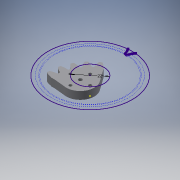
# Autodesk Inventor part: ENGE
Saved by Autodesk Inventor 2017 (Build 210142000, 142)
## iProperties
Created: 2018-01-13
Part Number: ENGE
Material: Generic
Document SubType Name: Modeling
Designer: Thomas
Density: 1 g/cm^3
Appearance: Default
Author: Thomas
Autodesk Inventor part; units mm, degrees
ref_plane "YZ Plane" through (0, 0, 0) normal (1, 0, 0) x (0, 1, 0)
ref_plane "XZ Plane" through (0, 0, 0) normal (0, 1, 0) x (-1, 0, 0)
ref_plane "XY Plane" through (0, 0, 0) normal (0, 0, 1) x (1, 0, 0)
sketch "Sketch1" plane through (0, 0, 0) normal (0, 0, 1) x (1, 0, 0)
  spline S0 degree 3 poles (-3.069, 32.857) (-2.9961, 32.7532) (-2.8503, 32.5455) (-2.641, 32.2277) (-2.4393, 31.9049) (-2.2462, 31.577) (-2.0623, 31.2438) (-1.8883, 30.9052) (-1.7251, 30.5614) (-1.5739, 30.2121) (-1.4358, 29.8574) (-1.3139, 29.4969) (-1.2064, 29.1316) (-1.1476, 28.8193) (-1.0633, 28.5794) (-0.9771, 28.4092) (-0.8642, 28.2551) (-0.725, 28.1239) (-0.5884, 28.0413) (-0.471, 27.9927) (-0.379, 27.968) (-0.2855, 27.9491) (-0.1585, 27.9444) (0, 27.9474) (0.1585, 27.9444) (0.2855, 27.9491) (0.379, 27.968) (0.471, 27.9927) (0.5884, 28.0413) (0.725, 28.1239) (0.8642, 28.2551) (0.9771, 28.4092) (1.0633, 28.5794) (1.1476, 28.8193) (1.2064, 29.1316) (1.3139, 29.4969) (1.4358, 29.8574) (1.5739, 30.2121) (1.7251, 30.5614) (1.8883, 30.9052) (2.0623, 31.2438) (2.2462, 31.577) (2.4393, 31.9049) (2.641, 32.2277) (2.8503, 32.5455) (2.9961, 32.7532) (3.069, 32.857) knots 0 0 0 0 0.038054 0.076108 0.114163 0.152217 0.190271 0.228324 0.266378 0.304431 0.342484 0.380536 0.418586 0.456634 0.47565 0.49466 0.513668 0.532673 0.551678 0.561193 0.570705 0.580215 0.589727 0.608754 0.627782 0.637294 0.646804 0.656316 0.66583 0.684836 0.703841 0.722849 0.741859 0.760875 0.798923 0.836973 0.875025 0.913077 0.95113 0.989184 1.027238 1.065292 1.103346 1.1414 1.179454 1.217508 1.217508 1.217508 1.217508
  circle A0 centre (0, 0) radius 27.9462 construction
  circle A1 centre (0, 0) radius 28.5432 construction
  circle A2 centre (0, 0) radius 30.375 construction
  circle A3 centre (0, 0) radius 33
  circle A4 centre (0, 0) radius 11
  point P0 (-2.8519, 32.5444)
  point P1 (-2.6423, 32.2269)
  point P2 (-2.4407, 31.9041)
  point P3 (-2.2477, 31.5761)
  point P4 (-2.0639, 31.2429)
  point P5 (-1.8901, 30.9044)
  point P6 (-1.7271, 30.5605)
  point P7 (-1.5761, 30.2112)
  point P8 (-1.4385, 29.8564)
  point P9 (-1.3163, 29.4961)
  point P10 (-1.2126, 29.13)
  point P11 (-1.1234, 28.7601)
  point P12 (-1.0595, 28.581)
  point P13 (-0.9726, 28.4119)
  point P14 (-0.8598, 28.2589)
  point P15 (-0.7209, 28.1293)
  point P16 (-0.5584, 28.0306)
  point P17 (-0.4703, 27.9947)
  point P18 (-0.3787, 27.969)
  point P19 (-0.2852, 27.9516)
  point P20 (-0.1903, 27.9462)
  point P21 (0, 27.9462)
  point P22 (0.1903, 27.9462)
  point P23 (0.2852, 27.9516)
  point P24 (0.3787, 27.969)
  point P25 (0.4703, 27.9947)
  point P26 (0.5584, 28.0306)
  point P27 (0.7209, 28.1293)
  point P28 (0.8598, 28.2589)
  point P29 (0.9726, 28.4119)
  point P30 (1.0595, 28.581)
  point P31 (1.1234, 28.7601)
  point P32 (1.2126, 29.13)
  point P33 (1.3163, 29.4961)
  point P34 (1.4385, 29.8564)
  point P35 (1.5761, 30.2112)
  point P36 (1.7271, 30.5605)
  point P37 (1.8901, 30.9044)
  point P38 (2.0639, 31.2429)
  point P39 (2.2477, 31.5761)
  point P40 (2.4407, 31.9041)
  point P41 (2.6423, 32.2269)
  point P42 (2.8519, 32.5444)
  dimension "d23" = 22
  constraints: 5 centre point, 2 point on circle, 1 coincident, 95 other
  measures "d23" diameter of A4
extrude "Extrusion1" add sketch "Sketch1" against normal blind 20 contours A3 S0 | S0 A3 | A4
extrude "Extrusion2" cut sketch "Sketch1" against normal blind 26.5 contours A3 S0 picked at (-0.225, 31.2542)
pattern_circular "Réseau circulaire1" count 26 over 360 about axis through (0, 0, -10) along (0, 0, 1) of "Extrusion2"
sketch "Esquisse2" plane through (0, 0, 0) normal (0, 0, 1) x (1, 0, 0)
  spline S0 degree 3 poles (28.7842, 16.1392) (28.6573, 16.1402) (28.4036, 16.1422) (28.0231, 16.1339) (27.6429, 16.1166) (27.2633, 16.0892) (26.8846, 16.0512) (26.5072, 16.0021) (26.1315, 15.9411) (25.7582, 15.8671) (25.3878, 15.7793) (25.0218, 15.6749) (24.6601, 15.5557) (24.3697, 15.4268) (24.1244, 15.3599) (23.9354, 15.3342) (23.7444, 15.3395) (23.5574, 15.3796) (23.4118, 15.445) (23.3051, 15.5141) (23.2325, 15.5757) (23.1638, 15.6419) (23.0878, 15.7438) (23.0003, 15.8759) (22.9078, 16.0047) (22.8394, 16.1119) (22.8019, 16.1996) (22.77, 16.2893) (22.7433, 16.4135) (22.7337, 16.5728) (22.7625, 16.762) (22.8253, 16.9424) (22.9164, 17.1101) (23.0659, 17.3156) (23.2895, 17.5415) (23.5291, 17.8374) (23.7566, 18.1426) (23.97, 18.4577) (24.1716, 18.7806) (24.3618, 19.1102) (24.5416, 19.4457) (24.7113, 19.7863) (24.8716, 20.1315) (25.0226, 20.4809) (25.1652, 20.8337) (25.2533, 21.0717) (25.2974, 21.1906) knots 0 0 0 0 0.031256 0.062512 0.093767 0.125023 0.156279 0.187534 0.218789 0.250044 0.281299 0.312553 0.343805 0.375056 0.390675 0.406289 0.421901 0.43751 0.453121 0.460935 0.468748 0.476559 0.484372 0.5 0.515628 0.523441 0.531252 0.539065 0.546879 0.56249 0.578099 0.593711 0.609325 0.624944 0.656195 0.687447 0.718701 0.749956 0.781211 0.812466 0.843721 0.874977 0.906233 0.937488 0.968744 1 1 1 1 projected
  arc A0 (-3.069, 32.857) -> (-4.8834, 32.6367) centre (0, 0) ccw projected
  spline S1 degree 3 poles (3.069, 32.857) (2.9961, 32.7532) (2.8503, 32.5455) (2.641, 32.2277) (2.4393, 31.9049) (2.2462, 31.577) (2.0623, 31.2438) (1.8883, 30.9052) (1.7251, 30.5614) (1.5739, 30.2121) (1.4358, 29.8574) (1.3139, 29.4969) (1.2064, 29.1316) (1.1476, 28.8193) (1.0633, 28.5794) (0.9771, 28.4092) (0.8642, 28.2551) (0.725, 28.1239) (0.5884, 28.0413) (0.471, 27.9927) (0.379, 27.968) (0.2855, 27.9491) (0.1585, 27.9444) (0, 27.9474) (-0.1585, 27.9444) (-0.2855, 27.9491) (-0.379, 27.968) (-0.471, 27.9927) (-0.5884, 28.0413) (-0.725, 28.1239) (-0.8642, 28.2551) (-0.9771, 28.4092) (-1.0633, 28.5794) (-1.1476, 28.8193) (-1.2064, 29.1316) (-1.3139, 29.4969) (-1.4358, 29.8574) (-1.5739, 30.2121) (-1.7251, 30.5614) (-1.8883, 30.9052) (-2.0623, 31.2438) (-2.2462, 31.577) (-2.4393, 31.9049) (-2.641, 32.2277) (-2.8503, 32.5455) (-2.9961, 32.7532) (-3.069, 32.857) knots 0 0 0 0 0.031256 0.062512 0.093767 0.125023 0.156279 0.187534 0.218789 0.250044 0.281299 0.312553 0.343805 0.375056 0.390675 0.406289 0.421901 0.43751 0.453121 0.460935 0.468748 0.476559 0.484372 0.5 0.515628 0.523441 0.531252 0.539065 0.546879 0.56249 0.578099 0.593711 0.609325 0.624944 0.656195 0.687447 0.718701 0.749956 0.781211 0.812466 0.843721 0.874977 0.906233 0.937488 0.968744 1 1 1 1 projected
  spline S2 degree 3 poles (-4.8834, 32.6367) (-4.9293, 32.5184) (-5.0211, 32.2819) (-5.1483, 31.9232) (-5.267, 31.5616) (-5.3759, 31.1969) (-5.4748, 30.8294) (-5.5627, 30.4591) (-5.6388, 30.0862) (-5.7021, 29.7109) (-5.7513, 29.3334) (-5.7834, 28.9542) (-5.8003, 28.5738) (-5.7827, 28.2565) (-5.8071, 28.0034) (-5.8501, 27.8175) (-5.9228, 27.6409) (-6.0266, 27.4802) (-6.1394, 27.3673) (-6.2418, 27.292) (-6.3252, 27.246) (-6.4114, 27.2052) (-6.5337, 27.1704) (-6.6882, 27.1353) (-6.8414, 27.0945) (-6.9659, 27.0686) (-7.0612, 27.0646) (-7.1564, 27.0666) (-7.282, 27.0856) (-7.4344, 27.1332) (-7.601, 27.2272) (-7.7475, 27.3499) (-7.8719, 27.4945) (-8.0111, 27.7072) (-8.143, 27.9963) (-8.3347, 28.3253) (-8.5394, 28.6462) (-8.7584, 28.9575) (-8.9888, 29.2605) (-9.2296, 29.5553) (-9.4795, 29.8423) (-9.7378, 30.1218) (-10.0037, 30.3941) (-10.2768, 30.6592) (-10.5562, 30.9177) (-10.7474, 31.0844) (-10.843, 31.1678) knots 0 0 0 0 0.031256 0.062512 0.093767 0.125023 0.156279 0.187534 0.218789 0.250044 0.281299 0.312553 0.343805 0.375056 0.390675 0.406289 0.421901 0.43751 0.453121 0.460935 0.468748 0.476559 0.484372 0.5 0.515628 0.523441 0.531252 0.539065 0.546879 0.56249 0.578099 0.593711 0.609325 0.624944 0.656195 0.687447 0.718701 0.749956 0.781211 0.812466 0.843721 0.874977 0.906233 0.937488 0.968744 1 1 1 1 projected
  arc A1 (-10.843, 31.1678) -> (-12.5519, 30.5196) centre (0, 0) ccw projected
  spline S3 degree 3 poles (-12.5519, 30.5196) (-12.5682, 30.3938) (-12.6008, 30.1422) (-12.6385, 29.7635) (-12.6671, 29.384) (-12.6856, 29.0039) (-12.6936, 28.6234) (-12.6904, 28.2428) (-12.6751, 27.8625) (-12.6466, 27.4829) (-12.6041, 27.1047) (-12.5445, 26.7288) (-12.4699, 26.3554) (-12.3769, 26.0515) (-12.34, 25.8) (-12.3373, 25.6092) (-12.3656, 25.4203) (-12.4279, 25.2394) (-12.5104, 25.1028) (-12.5918, 25.0052) (-12.6618, 24.9406) (-12.7357, 24.8804) (-12.8461, 24.8172) (-12.9878, 24.7462) (-13.1268, 24.6699) (-13.2414, 24.615) (-13.333, 24.5883) (-13.4259, 24.5674) (-13.5524, 24.5559) (-13.7118, 24.5656) (-13.896, 24.617) (-14.0676, 24.7011) (-14.223, 24.8117) (-14.4091, 24.9849) (-14.6064, 25.2341) (-14.8712, 25.5076) (-15.1467, 25.7702) (-15.4339, 26.0201) (-15.7301, 26.2591) (-16.0344, 26.4877) (-16.3458, 26.7066) (-16.6635, 26.9161) (-16.9868, 27.1168) (-17.3154, 27.3089) (-17.6485, 27.493) (-17.8741, 27.6091) (-17.9869, 27.6672) knots 0 0 0 0 0.031256 0.062512 0.093767 0.125023 0.156279 0.187534 0.218789 0.250044 0.281299 0.312553 0.343805 0.375056 0.390675 0.406289 0.421901 0.43751 0.453121 0.460935 0.468748 0.476559 0.484372 0.5 0.515628 0.523441 0.531252 0.539065 0.546879 0.56249 0.578099 0.593711 0.609325 0.624944 0.656195 0.687447 0.718701 0.749956 0.781211 0.812466 0.843721 0.874977 0.906233 0.937488 0.968744 1 1 1 1 projected
  arc A2 (-17.9869, 27.6672) -> (-19.491, 26.6289) centre (0, 0) ccw projected
  spline S4 degree 3 poles (-19.491, 26.6289) (-19.4767, 26.5029) (-19.4482, 26.2508) (-19.3941, 25.874) (-19.3311, 25.4987) (-19.2581, 25.1252) (-19.1748, 24.7538) (-19.0805, 24.3851) (-18.9747, 24.0195) (-18.8562, 23.6578) (-18.7244, 23.3007) (-18.5766, 22.95) (-18.4148, 22.6053) (-18.2518, 22.3325) (-18.1558, 22.0971) (-18.1075, 21.9125) (-18.0897, 21.7223) (-18.107, 21.5318) (-18.1544, 21.3794) (-18.2101, 21.2652) (-18.2625, 21.1857) (-18.3199, 21.1095) (-18.412, 21.0218) (-18.5325, 20.9189) (-18.6492, 20.8116) (-18.7474, 20.7308) (-18.8299, 20.683) (-18.9151, 20.6405) (-19.0352, 20.599) (-19.1923, 20.5703) (-19.3835, 20.5762) (-19.5702, 20.6167) (-19.7476, 20.6869) (-19.9697, 20.8106) (-20.2208, 21.0053) (-20.5435, 21.2075) (-20.8738, 21.3965) (-21.2124, 21.5704) (-21.5572, 21.7316) (-21.9074, 21.8807) (-22.2621, 22.0187) (-22.6207, 22.1462) (-22.9827, 22.2637) (-23.3477, 22.3715) (-23.7152, 22.4705) (-23.962, 22.5293) (-24.0854, 22.5587) knots 0 0 0 0 0.031256 0.062512 0.093767 0.125023 0.156279 0.187534 0.218789 0.250044 0.281299 0.312553 0.343805 0.375056 0.390675 0.406289 0.421901 0.43751 0.453121 0.460935 0.468748 0.476559 0.484372 0.5 0.515628 0.523441 0.531252 0.539065 0.546879 0.56249 0.578099 0.593711 0.609325 0.624944 0.656195 0.687447 0.718701 0.749956 0.781211 0.812466 0.843721 0.874977 0.906233 0.937488 0.968744 1 1 1 1 projected
  arc A3 (-24.0854, 22.5587) -> (-25.2974, 21.1906) centre (0, 0) ccw projected
  spline S5 degree 3 poles (-25.2974, 21.1906) (-25.2533, 21.0717) (-25.1652, 20.8337) (-25.0226, 20.4809) (-24.8716, 20.1315) (-24.7113, 19.7863) (-24.5416, 19.4457) (-24.3618, 19.1102) (-24.1716, 18.7806) (-23.97, 18.4577) (-23.7566, 18.1426) (-23.5291, 17.8374) (-23.2895, 17.5415) (-23.0659, 17.3156) (-22.9164, 17.1101) (-22.8253, 16.9424) (-22.7625, 16.762) (-22.7337, 16.5728) (-22.7433, 16.4135) (-22.77, 16.2893) (-22.8019, 16.1996) (-22.8394, 16.1119) (-22.9078, 16.0047) (-23.0003, 15.8759) (-23.0878, 15.7438) (-23.1638, 15.6419) (-23.2325, 15.5757) (-23.3051, 15.5141) (-23.4118, 15.445) (-23.5574, 15.3796) (-23.7444, 15.3395) (-23.9354, 15.3342) (-24.1244, 15.3599) (-24.3697, 15.4268) (-24.6601, 15.5557) (-25.0218, 15.6749) (-25.3878, 15.7793) (-25.7582, 15.8671) (-26.1315, 15.9411) (-26.5072, 16.0021) (-26.8846, 16.0512) (-27.2633, 16.0892) (-27.6429, 16.1166) (-28.0231, 16.1339) (-28.4036, 16.1422) (-28.6573, 16.1402) (-28.7842, 16.1392) knots 0 0 0 0 0.031256 0.062512 0.093767 0.125023 0.156279 0.187534 0.218789 0.250044 0.281299 0.312553 0.343805 0.375056 0.390675 0.406289 0.421901 0.43751 0.453121 0.460935 0.468748 0.476559 0.484372 0.5 0.515628 0.523441 0.531252 0.539065 0.546879 0.56249 0.578099 0.593711 0.609325 0.624944 0.656195 0.687447 0.718701 0.749956 0.781211 0.812466 0.843721 0.874977 0.906233 0.937488 0.968744 1 1 1 1 projected
  arc A4 (-28.7842, 16.1392) -> (-29.6335, 14.5208) centre (0, 0) ccw projected
  spline S6 degree 3 poles (-29.6335, 14.5208) (-29.5623, 14.4158) (-29.4198, 14.2059) (-29.1969, 13.8974) (-28.9667, 13.5944) (-28.7285, 13.2976) (-28.4821, 13.0075) (-28.2273, 12.7248) (-27.9637, 12.4502) (-27.6907, 12.185) (-27.408, 11.9301) (-27.1142, 11.6882) (-26.8107, 11.4582) (-26.5396, 11.2924) (-26.3452, 11.1286) (-26.2166, 10.9876) (-26.1125, 10.8275) (-26.0392, 10.6507) (-26.0104, 10.4937) (-26.0066, 10.3667) (-26.0162, 10.272) (-26.0316, 10.1779) (-26.0723, 10.0574) (-26.1313, 9.9103) (-26.1847, 9.7611) (-26.2341, 9.6439) (-26.2849, 9.5632) (-26.3407, 9.486) (-26.4277, 9.3934) (-26.5534, 9.295) (-26.7254, 9.2113) (-26.9096, 9.1605) (-27.0993, 9.1402) (-27.3534, 9.1465) (-27.6663, 9.2022) (-28.046, 9.2313) (-28.4263, 9.2451) (-28.8069, 9.2417) (-29.1871, 9.2242) (-29.5665, 9.1935) (-29.9447, 9.1509) (-30.3215, 9.0971) (-30.6966, 9.0329) (-31.0699, 8.9587) (-31.4413, 8.8757) (-31.6872, 8.813) (-31.8101, 8.7817) knots 0 0 0 0 0.031256 0.062512 0.093767 0.125023 0.156279 0.187534 0.218789 0.250044 0.281299 0.312553 0.343805 0.375056 0.390675 0.406289 0.421901 0.43751 0.453121 0.460935 0.468748 0.476559 0.484372 0.5 0.515628 0.523441 0.531252 0.539065 0.546879 0.56249 0.578099 0.593711 0.609325 0.624944 0.656195 0.687447 0.718701 0.749956 0.781211 0.812466 0.843721 0.874977 0.906233 0.937488 0.968744 1 1 1 1 projected
  arc A5 (-31.8101, 8.7817) -> (-32.2475, 7.0071) centre (0, 0) ccw projected
  spline S7 degree 3 poles (-32.2475, 7.0071) (-32.1532, 6.9222) (-31.9646, 6.7525) (-31.6744, 6.5063) (-31.3783, 6.2672) (-31.076, 6.036) (-30.7674, 5.8133) (-30.4523, 5.5998) (-30.1306, 5.3963) (-29.8021, 5.2041) (-29.4667, 5.0242) (-29.1235, 4.8597) (-28.7738, 4.7091) (-28.4708, 4.613) (-28.2429, 4.5004) (-28.0843, 4.3943) (-27.9449, 4.2637) (-27.8315, 4.1096) (-27.7659, 3.9641) (-27.7318, 3.8417) (-27.7184, 3.7474) (-27.7109, 3.6523) (-27.7216, 3.5257) (-27.7436, 3.3687) (-27.7598, 3.211) (-27.7797, 3.0854) (-27.8098, 2.9949) (-27.8454, 2.9066) (-27.9078, 2.7959) (-28.0062, 2.6703) (-28.1533, 2.5478) (-28.3199, 2.4544) (-28.4992, 2.3893) (-28.7475, 2.3346) (-29.0646, 2.3138) (-29.4402, 2.2512) (-29.8128, 2.1736) (-30.1816, 2.0792) (-30.5465, 1.9712) (-30.9075, 1.8507) (-31.2645, 1.7188) (-31.6175, 1.5764) (-31.9663, 1.4242) (-32.311, 1.2629) (-32.6518, 1.0934) (-32.8755, 0.9737) (-32.9873, 0.9139) knots 0 0 0 0 0.031256 0.062512 0.093767 0.125023 0.156279 0.187534 0.218789 0.250044 0.281299 0.312553 0.343805 0.375056 0.390675 0.406289 0.421901 0.43751 0.453121 0.460935 0.468748 0.476559 0.484372 0.5 0.515628 0.523441 0.531252 0.539065 0.546879 0.56249 0.578099 0.593711 0.609325 0.624944 0.656195 0.687447 0.718701 0.749956 0.781211 0.812466 0.843721 0.874977 0.906233 0.937488 0.968744 1 1 1 1 projected
  arc A6 (-32.9873, 0.9139) -> (-32.9873, -0.9139) centre (0, 0) ccw projected
  spline S8 degree 3 poles (-32.9873, -0.9139) (-32.8755, -0.9737) (-32.6518, -1.0934) (-32.311, -1.2629) (-31.9663, -1.4242) (-31.6175, -1.5764) (-31.2645, -1.7188) (-30.9075, -1.8507) (-30.5465, -1.9712) (-30.1816, -2.0792) (-29.8128, -2.1736) (-29.4402, -2.2512) (-29.0646, -2.3138) (-28.7475, -2.3346) (-28.4992, -2.3893) (-28.3199, -2.4544) (-28.1533, -2.5478) (-28.0062, -2.6703) (-27.9078, -2.7959) (-27.8454, -2.9066) (-27.8098, -2.9949) (-27.7797, -3.0854) (-27.7598, -3.211) (-27.7436, -3.3687) (-27.7216, -3.5257) (-27.7109, -3.6523) (-27.7184, -3.7474) (-27.7318, -3.8417) (-27.7659, -3.9641) (-27.8315, -4.1096) (-27.9449, -4.2637) (-28.0843, -4.3943) (-28.2429, -4.5004) (-28.4708, -4.613) (-28.7738, -4.7091) (-29.1235, -4.8597) (-29.4667, -5.0242) (-29.8021, -5.2041) (-30.1306, -5.3963) (-30.4523, -5.5998) (-30.7674, -5.8133) (-31.076, -6.036) (-31.3783, -6.2672) (-31.6744, -6.5063) (-31.9646, -6.7525) (-32.1532, -6.9222) (-32.2475, -7.0071) knots 0 0 0 0 0.031256 0.062512 0.093767 0.125023 0.156279 0.187534 0.218789 0.250044 0.281299 0.312553 0.343805 0.375056 0.390675 0.406289 0.421901 0.43751 0.453121 0.460935 0.468748 0.476559 0.484372 0.5 0.515628 0.523441 0.531252 0.539065 0.546879 0.56249 0.578099 0.593711 0.609325 0.624944 0.656195 0.687447 0.718701 0.749956 0.781211 0.812466 0.843721 0.874977 0.906233 0.937488 0.968744 1 1 1 1 projected
  arc A7 (-32.2475, -7.0071) -> (-31.8101, -8.7817) centre (0, 0) ccw projected
  spline S9 degree 3 poles (-31.8101, -8.7817) (-31.6872, -8.813) (-31.4413, -8.8757) (-31.0699, -8.9587) (-30.6966, -9.0329) (-30.3215, -9.0971) (-29.9447, -9.1509) (-29.5665, -9.1935) (-29.1871, -9.2242) (-28.8069, -9.2417) (-28.4263, -9.2451) (-28.046, -9.2313) (-27.6663, -9.2022) (-27.3534, -9.1465) (-27.0993, -9.1402) (-26.9096, -9.1605) (-26.7254, -9.2113) (-26.5534, -9.295) (-26.4277, -9.3934) (-26.3407, -9.486) (-26.2849, -9.5632) (-26.2341, -9.6439) (-26.1847, -9.7611) (-26.1313, -9.9103) (-26.0723, -10.0574) (-26.0316, -10.1779) (-26.0162, -10.272) (-26.0066, -10.3667) (-26.0104, -10.4937) (-26.0392, -10.6507) (-26.1125, -10.8275) (-26.2166, -10.9876) (-26.3452, -11.1286) (-26.5396, -11.2924) (-26.8107, -11.4582) (-27.1142, -11.6882) (-27.408, -11.9301) (-27.6907, -12.185) (-27.9637, -12.4502) (-28.2273, -12.7248) (-28.4821, -13.0075) (-28.7285, -13.2976) (-28.9667, -13.5944) (-29.1969, -13.8974) (-29.4198, -14.2059) (-29.5623, -14.4158) (-29.6335, -14.5208) knots 0 0 0 0 0.031256 0.062512 0.093767 0.125023 0.156279 0.187534 0.218789 0.250044 0.281299 0.312553 0.343805 0.375056 0.390675 0.406289 0.421901 0.43751 0.453121 0.460935 0.468748 0.476559 0.484372 0.5 0.515628 0.523441 0.531252 0.539065 0.546879 0.56249 0.578099 0.593711 0.609325 0.624944 0.656195 0.687447 0.718701 0.749956 0.781211 0.812466 0.843721 0.874977 0.906233 0.937488 0.968744 1 1 1 1 projected
  arc A8 (-29.6335, -14.5208) -> (-28.7842, -16.1392) centre (0, 0) ccw projected
  spline S10 degree 3 poles (-28.7842, -16.1392) (-28.6573, -16.1402) (-28.4036, -16.1422) (-28.0231, -16.1339) (-27.6429, -16.1166) (-27.2633, -16.0892) (-26.8846, -16.0512) (-26.5072, -16.0021) (-26.1315, -15.9411) (-25.7582, -15.8671) (-25.3878, -15.7793) (-25.0218, -15.6749) (-24.6601, -15.5557) (-24.3697, -15.4268) (-24.1244, -15.3599) (-23.9354, -15.3342) (-23.7444, -15.3395) (-23.5574, -15.3796) (-23.4118, -15.445) (-23.3051, -15.5141) (-23.2325, -15.5757) (-23.1638, -15.6419) (-23.0878, -15.7438) (-23.0003, -15.8759) (-22.9078, -16.0047) (-22.8394, -16.1119) (-22.8019, -16.1996) (-22.77, -16.2893) (-22.7433, -16.4135) (-22.7337, -16.5728) (-22.7625, -16.762) (-22.8253, -16.9424) (-22.9164, -17.1101) (-23.0659, -17.3156) (-23.2895, -17.5415) (-23.5291, -17.8374) (-23.7566, -18.1426) (-23.97, -18.4577) (-24.1716, -18.7806) (-24.3618, -19.1102) (-24.5416, -19.4457) (-24.7113, -19.7863) (-24.8716, -20.1315) (-25.0226, -20.4809) (-25.1652, -20.8337) (-25.2533, -21.0717) (-25.2974, -21.1906) knots 0 0 0 0 0.031256 0.062512 0.093767 0.125023 0.156279 0.187534 0.218789 0.250044 0.281299 0.312553 0.343805 0.375056 0.390675 0.406289 0.421901 0.43751 0.453121 0.460935 0.468748 0.476559 0.484372 0.5 0.515628 0.523441 0.531252 0.539065 0.546879 0.56249 0.578099 0.593711 0.609325 0.624944 0.656195 0.687447 0.718701 0.749956 0.781211 0.812466 0.843721 0.874977 0.906233 0.937488 0.968744 1 1 1 1 projected
  arc A9 (-25.2974, -21.1906) -> (-24.0854, -22.5587) centre (0, 0) ccw projected
  spline S11 degree 3 poles (-24.0854, -22.5587) (-23.962, -22.5293) (-23.7152, -22.4705) (-23.3477, -22.3715) (-22.9827, -22.2637) (-22.6207, -22.1462) (-22.2621, -22.0187) (-21.9074, -21.8807) (-21.5572, -21.7316) (-21.2124, -21.5704) (-20.8738, -21.3965) (-20.5435, -21.2075) (-20.2208, -21.0053) (-19.9697, -20.8106) (-19.7476, -20.6869) (-19.5702, -20.6167) (-19.3835, -20.5762) (-19.1923, -20.5703) (-19.0352, -20.599) (-18.9151, -20.6405) (-18.8299, -20.683) (-18.7474, -20.7308) (-18.6492, -20.8116) (-18.5325, -20.9189) (-18.412, -21.0218) (-18.3199, -21.1095) (-18.2625, -21.1857) (-18.2101, -21.2652) (-18.1544, -21.3794) (-18.107, -21.5318) (-18.0897, -21.7223) (-18.1075, -21.9125) (-18.1558, -22.0971) (-18.2518, -22.3325) (-18.4148, -22.6053) (-18.5766, -22.95) (-18.7244, -23.3007) (-18.8562, -23.6578) (-18.9747, -24.0195) (-19.0805, -24.3851) (-19.1748, -24.7538) (-19.2581, -25.1252) (-19.3311, -25.4987) (-19.3941, -25.874) (-19.4482, -26.2508) (-19.4767, -26.5029) (-19.491, -26.6289) knots 0 0 0 0 0.031256 0.062512 0.093767 0.125023 0.156279 0.187534 0.218789 0.250044 0.281299 0.312553 0.343805 0.375056 0.390675 0.406289 0.421901 0.43751 0.453121 0.460935 0.468748 0.476559 0.484372 0.5 0.515628 0.523441 0.531252 0.539065 0.546879 0.56249 0.578099 0.593711 0.609325 0.624944 0.656195 0.687447 0.718701 0.749956 0.781211 0.812466 0.843721 0.874977 0.906233 0.937488 0.968744 1 1 1 1 projected
  arc A10 (-19.491, -26.6289) -> (-17.9869, -27.6672) centre (0, 0) ccw projected
  spline S12 degree 3 poles (-17.9869, -27.6672) (-17.8741, -27.6091) (-17.6485, -27.493) (-17.3154, -27.3089) (-16.9868, -27.1168) (-16.6635, -26.9161) (-16.3458, -26.7066) (-16.0344, -26.4877) (-15.7301, -26.2591) (-15.4339, -26.0201) (-15.1467, -25.7702) (-14.8712, -25.5076) (-14.6064, -25.2341) (-14.4091, -24.9849) (-14.223, -24.8117) (-14.0676, -24.7011) (-13.896, -24.617) (-13.7118, -24.5656) (-13.5524, -24.5559) (-13.4259, -24.5674) (-13.333, -24.5883) (-13.2414, -24.615) (-13.1268, -24.6699) (-12.9878, -24.7462) (-12.8461, -24.8172) (-12.7357, -24.8804) (-12.6618, -24.9406) (-12.5918, -25.0052) (-12.5104, -25.1028) (-12.4279, -25.2394) (-12.3656, -25.4203) (-12.3373, -25.6092) (-12.34, -25.8) (-12.3769, -26.0515) (-12.4699, -26.3554) (-12.5445, -26.7288) (-12.6041, -27.1047) (-12.6466, -27.4829) (-12.6751, -27.8625) (-12.6904, -28.2428) (-12.6936, -28.6234) (-12.6856, -29.0039) (-12.6671, -29.384) (-12.6385, -29.7635) (-12.6008, -30.1422) (-12.5682, -30.3938) (-12.5519, -30.5196) knots 0 0 0 0 0.031256 0.062512 0.093767 0.125023 0.156279 0.187534 0.218789 0.250044 0.281299 0.312553 0.343805 0.375056 0.390675 0.406289 0.421901 0.43751 0.453121 0.460935 0.468748 0.476559 0.484372 0.5 0.515628 0.523441 0.531252 0.539065 0.546879 0.56249 0.578099 0.593711 0.609325 0.624944 0.656195 0.687447 0.718701 0.749956 0.781211 0.812466 0.843721 0.874977 0.906233 0.937488 0.968744 1 1 1 1 projected
  arc A11 (-12.5519, -30.5196) -> (-10.843, -31.1678) centre (0, 0) ccw projected
  spline S13 degree 3 poles (-10.843, -31.1678) (-10.7474, -31.0844) (-10.5562, -30.9177) (-10.2768, -30.6592) (-10.0037, -30.3941) (-9.7378, -30.1218) (-9.4795, -29.8423) (-9.2296, -29.5553) (-8.9888, -29.2605) (-8.7584, -28.9575) (-8.5394, -28.6462) (-8.3347, -28.3253) (-8.143, -27.9963) (-8.0111, -27.7072) (-7.8719, -27.4945) (-7.7475, -27.3499) (-7.601, -27.2272) (-7.4344, -27.1332) (-7.282, -27.0856) (-7.1564, -27.0666) (-7.0612, -27.0646) (-6.9659, -27.0686) (-6.8414, -27.0945) (-6.6882, -27.1353) (-6.5337, -27.1704) (-6.4114, -27.2052) (-6.3252, -27.246) (-6.2418, -27.292) (-6.1394, -27.3673) (-6.0266, -27.4802) (-5.9228, -27.6409) (-5.8501, -27.8175) (-5.8071, -28.0034) (-5.7827, -28.2565) (-5.8003, -28.5738) (-5.7834, -28.9542) (-5.7513, -29.3334) (-5.7021, -29.7109) (-5.6388, -30.0862) (-5.5627, -30.4591) (-5.4748, -30.8294) (-5.3759, -31.1969) (-5.267, -31.5616) (-5.1483, -31.9232) (-5.0211, -32.2819) (-4.9293, -32.5184) (-4.8834, -32.6367) knots 0 0 0 0 0.031256 0.062512 0.093767 0.125023 0.156279 0.187534 0.218789 0.250044 0.281299 0.312553 0.343805 0.375056 0.390675 0.406289 0.421901 0.43751 0.453121 0.460935 0.468748 0.476559 0.484372 0.5 0.515628 0.523441 0.531252 0.539065 0.546879 0.56249 0.578099 0.593711 0.609325 0.624944 0.656195 0.687447 0.718701 0.749956 0.781211 0.812466 0.843721 0.874977 0.906233 0.937488 0.968744 1 1 1 1 projected
  arc A12 (-4.8834, -32.6367) -> (-3.069, -32.857) centre (0, 0) ccw projected
  spline S14 degree 3 poles (-3.069, -32.857) (-2.9961, -32.7532) (-2.8503, -32.5455) (-2.641, -32.2277) (-2.4393, -31.9049) (-2.2462, -31.577) (-2.0623, -31.2438) (-1.8883, -30.9052) (-1.7251, -30.5614) (-1.5739, -30.2121) (-1.4358, -29.8574) (-1.3139, -29.4969) (-1.2064, -29.1316) (-1.1476, -28.8193) (-1.0633, -28.5794) (-0.9771, -28.4092) (-0.8642, -28.2551) (-0.725, -28.1239) (-0.5884, -28.0413) (-0.471, -27.9927) (-0.379, -27.968) (-0.2855, -27.9491) (-0.1585, -27.9444) (0, -27.9474) (0.1585, -27.9444) (0.2855, -27.9491) (0.379, -27.968) (0.471, -27.9927) (0.5884, -28.0413) (0.725, -28.1239) (0.8642, -28.2551) (0.9771, -28.4092) (1.0633, -28.5794) (1.1476, -28.8193) (1.2064, -29.1316) (1.3139, -29.4969) (1.4358, -29.8574) (1.5739, -30.2121) (1.7251, -30.5614) (1.8883, -30.9052) (2.0623, -31.2438) (2.2462, -31.577) (2.4393, -31.9049) (2.641, -32.2277) (2.8503, -32.5455) (2.9961, -32.7532) (3.069, -32.857) knots 0 0 0 0 0.031256 0.062512 0.093767 0.125023 0.156279 0.187534 0.218789 0.250044 0.281299 0.312553 0.343805 0.375056 0.390675 0.406289 0.421901 0.43751 0.453121 0.460935 0.468748 0.476559 0.484372 0.5 0.515628 0.523441 0.531252 0.539065 0.546879 0.56249 0.578099 0.593711 0.609325 0.624944 0.656195 0.687447 0.718701 0.749956 0.781211 0.812466 0.843721 0.874977 0.906233 0.937488 0.968744 1 1 1 1 projected
  arc A13 (3.069, -32.857) -> (4.8834, -32.6367) centre (0, 0) ccw projected
  spline S15 degree 3 poles (4.8834, -32.6367) (4.9293, -32.5184) (5.0211, -32.2819) (5.1483, -31.9232) (5.267, -31.5616) (5.3759, -31.1969) (5.4748, -30.8294) (5.5627, -30.4591) (5.6388, -30.0862) (5.7021, -29.7109) (5.7513, -29.3334) (5.7834, -28.9542) (5.8003, -28.5738) (5.7827, -28.2565) (5.8071, -28.0034) (5.8501, -27.8175) (5.9228, -27.6409) (6.0266, -27.4802) (6.1394, -27.3673) (6.2418, -27.292) (6.3252, -27.246) (6.4114, -27.2052) (6.5337, -27.1704) (6.6882, -27.1353) (6.8414, -27.0945) (6.9659, -27.0686) (7.0612, -27.0646) (7.1564, -27.0666) (7.282, -27.0856) (7.4344, -27.1332) (7.601, -27.2272) (7.7475, -27.3499) (7.8719, -27.4945) (8.0111, -27.7072) (8.143, -27.9963) (8.3347, -28.3253) (8.5394, -28.6462) (8.7584, -28.9575) (8.9888, -29.2605) (9.2296, -29.5553) (9.4795, -29.8423) (9.7378, -30.1218) (10.0037, -30.3941) (10.2768, -30.6592) (10.5562, -30.9177) (10.7474, -31.0844) (10.843, -31.1678) knots 0 0 0 0 0.031256 0.062512 0.093767 0.125023 0.156279 0.187534 0.218789 0.250044 0.281299 0.312553 0.343805 0.375056 0.390675 0.406289 0.421901 0.43751 0.453121 0.460935 0.468748 0.476559 0.484372 0.5 0.515628 0.523441 0.531252 0.539065 0.546879 0.56249 0.578099 0.593711 0.609325 0.624944 0.656195 0.687447 0.718701 0.749956 0.781211 0.812466 0.843721 0.874977 0.906233 0.937488 0.968744 1 1 1 1 projected
  arc A14 (10.843, -31.1678) -> (12.5519, -30.5196) centre (0, 0) ccw projected
  spline S16 degree 3 poles (12.5519, -30.5196) (12.5682, -30.3938) (12.6008, -30.1422) (12.6385, -29.7635) (12.6671, -29.384) (12.6856, -29.0039) (12.6936, -28.6234) (12.6904, -28.2428) (12.6751, -27.8625) (12.6466, -27.4829) (12.6041, -27.1047) (12.5445, -26.7288) (12.4699, -26.3554) (12.3769, -26.0515) (12.34, -25.8) (12.3373, -25.6092) (12.3656, -25.4203) (12.4279, -25.2394) (12.5104, -25.1028) (12.5918, -25.0052) (12.6618, -24.9406) (12.7357, -24.8804) (12.8461, -24.8172) (12.9878, -24.7462) (13.1268, -24.6699) (13.2414, -24.615) (13.333, -24.5883) (13.4259, -24.5674) (13.5524, -24.5559) (13.7118, -24.5656) (13.896, -24.617) (14.0676, -24.7011) (14.223, -24.8117) (14.4091, -24.9849) (14.6064, -25.2341) (14.8712, -25.5076) (15.1467, -25.7702) (15.4339, -26.0201) (15.7301, -26.2591) (16.0344, -26.4877) (16.3458, -26.7066) (16.6635, -26.9161) (16.9868, -27.1168) (17.3154, -27.3089) (17.6485, -27.493) (17.8741, -27.6091) (17.9869, -27.6672) knots 0 0 0 0 0.031256 0.062512 0.093767 0.125023 0.156279 0.187534 0.218789 0.250044 0.281299 0.312553 0.343805 0.375056 0.390675 0.406289 0.421901 0.43751 0.453121 0.460935 0.468748 0.476559 0.484372 0.5 0.515628 0.523441 0.531252 0.539065 0.546879 0.56249 0.578099 0.593711 0.609325 0.624944 0.656195 0.687447 0.718701 0.749956 0.781211 0.812466 0.843721 0.874977 0.906233 0.937488 0.968744 1 1 1 1 projected
  arc A15 (17.9869, -27.6672) -> (19.491, -26.6289) centre (0, 0) ccw projected
  spline S17 degree 3 poles (19.491, -26.6289) (19.4767, -26.5029) (19.4482, -26.2508) (19.3941, -25.874) (19.3311, -25.4987) (19.2581, -25.1252) (19.1748, -24.7538) (19.0805, -24.3851) (18.9747, -24.0195) (18.8562, -23.6578) (18.7244, -23.3007) (18.5766, -22.95) (18.4148, -22.6053) (18.2518, -22.3325) (18.1558, -22.0971) (18.1075, -21.9125) (18.0897, -21.7223) (18.107, -21.5318) (18.1544, -21.3794) (18.2101, -21.2652) (18.2625, -21.1857) (18.3199, -21.1095) (18.412, -21.0218) (18.5325, -20.9189) (18.6492, -20.8116) (18.7474, -20.7308) (18.8299, -20.683) (18.9151, -20.6405) (19.0352, -20.599) (19.1923, -20.5703) (19.3835, -20.5762) (19.5702, -20.6167) (19.7476, -20.6869) (19.9697, -20.8106) (20.2208, -21.0053) (20.5435, -21.2075) (20.8738, -21.3965) (21.2124, -21.5704) (21.5572, -21.7316) (21.9074, -21.8807) (22.2621, -22.0187) (22.6207, -22.1462) (22.9827, -22.2637) (23.3477, -22.3715) (23.7152, -22.4705) (23.962, -22.5293) (24.0854, -22.5587) knots 0 0 0 0 0.031256 0.062512 0.093767 0.125023 0.156279 0.187534 0.218789 0.250044 0.281299 0.312553 0.343805 0.375056 0.390675 0.406289 0.421901 0.43751 0.453121 0.460935 0.468748 0.476559 0.484372 0.5 0.515628 0.523441 0.531252 0.539065 0.546879 0.56249 0.578099 0.593711 0.609325 0.624944 0.656195 0.687447 0.718701 0.749956 0.781211 0.812466 0.843721 0.874977 0.906233 0.937488 0.968744 1 1 1 1 projected
  arc A16 (24.0854, -22.5587) -> (25.2974, -21.1906) centre (0, 0) ccw projected
  spline S18 degree 3 poles (25.2974, -21.1906) (25.2533, -21.0717) (25.1652, -20.8337) (25.0226, -20.4809) (24.8716, -20.1315) (24.7113, -19.7863) (24.5416, -19.4457) (24.3618, -19.1102) (24.1716, -18.7806) (23.97, -18.4577) (23.7566, -18.1426) (23.5291, -17.8374) (23.2895, -17.5415) (23.0659, -17.3156) (22.9164, -17.1101) (22.8253, -16.9424) (22.7625, -16.762) (22.7337, -16.5728) (22.7433, -16.4135) (22.77, -16.2893) (22.8019, -16.1996) (22.8394, -16.1119) (22.9078, -16.0047) (23.0003, -15.8759) (23.0878, -15.7438) (23.1638, -15.6419) (23.2325, -15.5757) (23.3051, -15.5141) (23.4118, -15.445) (23.5574, -15.3796) (23.7444, -15.3395) (23.9354, -15.3342) (24.1244, -15.3599) (24.3697, -15.4268) (24.6601, -15.5557) (25.0218, -15.6749) (25.3878, -15.7793) (25.7582, -15.8671) (26.1315, -15.9411) (26.5072, -16.0021) (26.8846, -16.0512) (27.2633, -16.0892) (27.6429, -16.1166) (28.0231, -16.1339) (28.4036, -16.1422) (28.6573, -16.1402) (28.7842, -16.1392) knots 0 0 0 0 0.031256 0.062512 0.093767 0.125023 0.156279 0.187534 0.218789 0.250044 0.281299 0.312553 0.343805 0.375056 0.390675 0.406289 0.421901 0.43751 0.453121 0.460935 0.468748 0.476559 0.484372 0.5 0.515628 0.523441 0.531252 0.539065 0.546879 0.56249 0.578099 0.593711 0.609325 0.624944 0.656195 0.687447 0.718701 0.749956 0.781211 0.812466 0.843721 0.874977 0.906233 0.937488 0.968744 1 1 1 1 projected
  arc A17 (28.7842, -16.1392) -> (29.6335, -14.5208) centre (0, 0) ccw projected
  spline S19 degree 3 poles (29.6335, -14.5208) (29.5623, -14.4158) (29.4198, -14.2059) (29.1969, -13.8974) (28.9667, -13.5944) (28.7285, -13.2976) (28.4821, -13.0075) (28.2273, -12.7248) (27.9637, -12.4502) (27.6907, -12.185) (27.408, -11.9301) (27.1142, -11.6882) (26.8107, -11.4582) (26.5396, -11.2924) (26.3452, -11.1286) (26.2166, -10.9876) (26.1125, -10.8275) (26.0392, -10.6507) (26.0104, -10.4937) (26.0066, -10.3667) (26.0162, -10.272) (26.0316, -10.1779) (26.0723, -10.0574) (26.1313, -9.9103) (26.1847, -9.7611) (26.2341, -9.6439) (26.2849, -9.5632) (26.3407, -9.486) (26.4277, -9.3934) (26.5534, -9.295) (26.7254, -9.2113) (26.9096, -9.1605) (27.0993, -9.1402) (27.3534, -9.1465) (27.6663, -9.2022) (28.046, -9.2313) (28.4263, -9.2451) (28.8069, -9.2417) (29.1871, -9.2242) (29.5665, -9.1935) (29.9447, -9.1509) (30.3215, -9.0971) (30.6966, -9.0329) (31.0699, -8.9587) (31.4413, -8.8757) (31.6872, -8.813) (31.8101, -8.7817) knots 0 0 0 0 0.031256 0.062512 0.093767 0.125023 0.156279 0.187534 0.218789 0.250044 0.281299 0.312553 0.343805 0.375056 0.390675 0.406289 0.421901 0.43751 0.453121 0.460935 0.468748 0.476559 0.484372 0.5 0.515628 0.523441 0.531252 0.539065 0.546879 0.56249 0.578099 0.593711 0.609325 0.624944 0.656195 0.687447 0.718701 0.749956 0.781211 0.812466 0.843721 0.874977 0.906233 0.937488 0.968744 1 1 1 1 projected
  arc A18 (31.8101, -8.7817) -> (32.2475, -7.0071) centre (0, 0) ccw projected
  spline S20 degree 3 poles (32.2475, -7.0071) (32.1532, -6.9222) (31.9646, -6.7525) (31.6744, -6.5063) (31.3783, -6.2672) (31.076, -6.036) (30.7674, -5.8133) (30.4523, -5.5998) (30.1306, -5.3963) (29.8021, -5.2041) (29.4667, -5.0242) (29.1235, -4.8597) (28.7738, -4.7091) (28.4708, -4.613) (28.2429, -4.5004) (28.0843, -4.3943) (27.9449, -4.2637) (27.8315, -4.1096) (27.7659, -3.9641) (27.7318, -3.8417) (27.7184, -3.7474) (27.7109, -3.6523) (27.7216, -3.5257) (27.7436, -3.3687) (27.7598, -3.211) (27.7797, -3.0854) (27.8098, -2.9949) (27.8454, -2.9066) (27.9078, -2.7959) (28.0062, -2.6703) (28.1533, -2.5478) (28.3199, -2.4544) (28.4992, -2.3893) (28.7475, -2.3346) (29.0646, -2.3138) (29.4402, -2.2512) (29.8128, -2.1736) (30.1816, -2.0792) (30.5465, -1.9712) (30.9075, -1.8507) (31.2645, -1.7188) (31.6175, -1.5764) (31.9663, -1.4242) (32.311, -1.2629) (32.6518, -1.0934) (32.8755, -0.9737) (32.9873, -0.9139) knots 0 0 0 0 0.031256 0.062512 0.093767 0.125023 0.156279 0.187534 0.218789 0.250044 0.281299 0.312553 0.343805 0.375056 0.390675 0.406289 0.421901 0.43751 0.453121 0.460935 0.468748 0.476559 0.484372 0.5 0.515628 0.523441 0.531252 0.539065 0.546879 0.56249 0.578099 0.593711 0.609325 0.624944 0.656195 0.687447 0.718701 0.749956 0.781211 0.812466 0.843721 0.874977 0.906233 0.937488 0.968744 1 1 1 1 projected
  arc A19 (32.9873, -0.9139) -> (32.9873, 0.9139) centre (0, 0) ccw projected
  spline S21 degree 3 poles (32.9873, 0.9139) (32.8755, 0.9737) (32.6518, 1.0934) (32.311, 1.2629) (31.9663, 1.4242) (31.6175, 1.5764) (31.2645, 1.7188) (30.9075, 1.8507) (30.5465, 1.9712) (30.1816, 2.0792) (29.8128, 2.1736) (29.4402, 2.2512) (29.0646, 2.3138) (28.7475, 2.3346) (28.4992, 2.3893) (28.3199, 2.4544) (28.1533, 2.5478) (28.0062, 2.6703) (27.9078, 2.7959) (27.8454, 2.9066) (27.8098, 2.9949) (27.7797, 3.0854) (27.7598, 3.211) (27.7436, 3.3687) (27.7216, 3.5257) (27.7109, 3.6523) (27.7184, 3.7474) (27.7318, 3.8417) (27.7659, 3.9641) (27.8315, 4.1096) (27.9449, 4.2637) (28.0843, 4.3943) (28.2429, 4.5004) (28.4708, 4.613) (28.7738, 4.7091) (29.1235, 4.8597) (29.4667, 5.0242) (29.8021, 5.2041) (30.1306, 5.3963) (30.4523, 5.5998) (30.7674, 5.8133) (31.076, 6.036) (31.3783, 6.2672) (31.6744, 6.5063) (31.9646, 6.7525) (32.1532, 6.9222) (32.2475, 7.0071) knots 0 0 0 0 0.031256 0.062512 0.093767 0.125023 0.156279 0.187534 0.218789 0.250044 0.281299 0.312553 0.343805 0.375056 0.390675 0.406289 0.421901 0.43751 0.453121 0.460935 0.468748 0.476559 0.484372 0.5 0.515628 0.523441 0.531252 0.539065 0.546879 0.56249 0.578099 0.593711 0.609325 0.624944 0.656195 0.687447 0.718701 0.749956 0.781211 0.812466 0.843721 0.874977 0.906233 0.937488 0.968744 1 1 1 1 projected
  arc A20 (32.2475, 7.0071) -> (31.8101, 8.7817) centre (0, 0) ccw projected
  spline S22 degree 3 poles (31.8101, 8.7817) (31.6872, 8.813) (31.4413, 8.8757) (31.0699, 8.9587) (30.6966, 9.0329) (30.3215, 9.0971) (29.9447, 9.1509) (29.5665, 9.1935) (29.1871, 9.2242) (28.8069, 9.2417) (28.4263, 9.2451) (28.046, 9.2313) (27.6663, 9.2022) (27.3534, 9.1465) (27.0993, 9.1402) (26.9096, 9.1605) (26.7254, 9.2113) (26.5534, 9.295) (26.4277, 9.3934) (26.3407, 9.486) (26.2849, 9.5632) (26.2341, 9.6439) (26.1847, 9.7611) (26.1313, 9.9103) (26.0723, 10.0574) (26.0316, 10.1779) (26.0162, 10.272) (26.0066, 10.3667) (26.0104, 10.4937) (26.0392, 10.6507) (26.1125, 10.8275) (26.2166, 10.9876) (26.3452, 11.1286) (26.5396, 11.2924) (26.8107, 11.4582) (27.1142, 11.6882) (27.408, 11.9301) (27.6907, 12.185) (27.9637, 12.4502) (28.2273, 12.7248) (28.4821, 13.0075) (28.7285, 13.2976) (28.9667, 13.5944) (29.1969, 13.8974) (29.4198, 14.2059) (29.5623, 14.4158) (29.6335, 14.5208) knots 0 0 0 0 0.031256 0.062512 0.093767 0.125023 0.156279 0.187534 0.218789 0.250044 0.281299 0.312553 0.343805 0.375056 0.390675 0.406289 0.421901 0.43751 0.453121 0.460935 0.468748 0.476559 0.484372 0.5 0.515628 0.523441 0.531252 0.539065 0.546879 0.56249 0.578099 0.593711 0.609325 0.624944 0.656195 0.687447 0.718701 0.749956 0.781211 0.812466 0.843721 0.874977 0.906233 0.937488 0.968744 1 1 1 1 projected
  arc A21 (29.6335, 14.5208) -> (28.7842, 16.1392) centre (0, 0) ccw projected
  spline S23 degree 3 poles (10.843, 31.1678) (10.7474, 31.0844) (10.5562, 30.9177) (10.2768, 30.6592) (10.0037, 30.3941) (9.7378, 30.1218) (9.4795, 29.8423) (9.2296, 29.5553) (8.9888, 29.2605) (8.7584, 28.9575) (8.5394, 28.6462) (8.3347, 28.3253) (8.143, 27.9963) (8.0111, 27.7072) (7.8719, 27.4945) (7.7475, 27.3499) (7.601, 27.2272) (7.4344, 27.1332) (7.282, 27.0856) (7.1564, 27.0666) (7.0612, 27.0646) (6.9659, 27.0686) (6.8414, 27.0945) (6.6882, 27.1353) (6.5337, 27.1704) (6.4114, 27.2052) (6.3252, 27.246) (6.2418, 27.292) (6.1394, 27.3673) (6.0266, 27.4802) (5.9228, 27.6409) (5.8501, 27.8175) (5.8071, 28.0034) (5.7827, 28.2565) (5.8003, 28.5738) (5.7834, 28.9542) (5.7513, 29.3334) (5.7021, 29.7109) (5.6388, 30.0862) (5.5627, 30.4591) (5.4748, 30.8294) (5.3759, 31.1969) (5.267, 31.5616) (5.1483, 31.9232) (5.0211, 32.2819) (4.9293, 32.5184) (4.8834, 32.6367) knots 0 0 0 0 0.031256 0.062512 0.093767 0.125023 0.156279 0.187534 0.218789 0.250044 0.281299 0.312553 0.343805 0.375056 0.390675 0.406289 0.421901 0.43751 0.453121 0.460935 0.468748 0.476559 0.484372 0.5 0.515628 0.523441 0.531252 0.539065 0.546879 0.56249 0.578099 0.593711 0.609325 0.624944 0.656195 0.687447 0.718701 0.749956 0.781211 0.812466 0.843721 0.874977 0.906233 0.937488 0.968744 1 1 1 1 projected
  arc A22 (4.8834, 32.6367) -> (3.069, 32.857) centre (0, 0) ccw projected
  arc A23 (25.2974, 21.1906) -> (24.0854, 22.5587) centre (0, 0) ccw projected
  spline S24 degree 3 poles (24.0854, 22.5587) (23.962, 22.5293) (23.7152, 22.4705) (23.3477, 22.3715) (22.9827, 22.2637) (22.6207, 22.1462) (22.2621, 22.0187) (21.9074, 21.8807) (21.5572, 21.7316) (21.2124, 21.5704) (20.8738, 21.3965) (20.5435, 21.2075) (20.2208, 21.0053) (19.9697, 20.8106) (19.7476, 20.6869) (19.5702, 20.6167) (19.3835, 20.5762) (19.1923, 20.5703) (19.0352, 20.599) (18.9151, 20.6405) (18.8299, 20.683) (18.7474, 20.7308) (18.6492, 20.8116) (18.5325, 20.9189) (18.412, 21.0218) (18.3199, 21.1095) (18.2625, 21.1857) (18.2101, 21.2652) (18.1544, 21.3794) (18.107, 21.5318) (18.0897, 21.7223) (18.1075, 21.9125) (18.1558, 22.0971) (18.2518, 22.3325) (18.4148, 22.6053) (18.5766, 22.95) (18.7244, 23.3007) (18.8562, 23.6578) (18.9747, 24.0195) (19.0805, 24.3851) (19.1748, 24.7538) (19.2581, 25.1252) (19.3311, 25.4987) (19.3941, 25.874) (19.4482, 26.2508) (19.4767, 26.5029) (19.491, 26.6289) knots 0 0 0 0 0.031256 0.062512 0.093767 0.125023 0.156279 0.187534 0.218789 0.250044 0.281299 0.312553 0.343805 0.375056 0.390675 0.406289 0.421901 0.43751 0.453121 0.460935 0.468748 0.476559 0.484372 0.5 0.515628 0.523441 0.531252 0.539065 0.546879 0.56249 0.578099 0.593711 0.609325 0.624944 0.656195 0.687447 0.718701 0.749956 0.781211 0.812466 0.843721 0.874977 0.906233 0.937488 0.968744 1 1 1 1 projected
  arc A24 (19.491, 26.6289) -> (17.9869, 27.6672) centre (0, 0) ccw projected
  spline S25 degree 3 poles (17.9869, 27.6672) (17.8741, 27.6091) (17.6485, 27.493) (17.3154, 27.3089) (16.9868, 27.1168) (16.6635, 26.9161) (16.3458, 26.7066) (16.0344, 26.4877) (15.7301, 26.2591) (15.4339, 26.0201) (15.1467, 25.7702) (14.8712, 25.5076) (14.6064, 25.2341) (14.4091, 24.9849) (14.223, 24.8117) (14.0676, 24.7011) (13.896, 24.617) (13.7118, 24.5656) (13.5524, 24.5559) (13.4259, 24.5674) (13.333, 24.5883) (13.2414, 24.615) (13.1268, 24.6699) (12.9878, 24.7462) (12.8461, 24.8172) (12.7357, 24.8804) (12.6618, 24.9406) (12.5918, 25.0052) (12.5104, 25.1028) (12.4279, 25.2394) (12.3656, 25.4203) (12.3373, 25.6092) (12.34, 25.8) (12.3769, 26.0515) (12.4699, 26.3554) (12.5445, 26.7288) (12.6041, 27.1047) (12.6466, 27.4829) (12.6751, 27.8625) (12.6904, 28.2428) (12.6936, 28.6234) (12.6856, 29.0039) (12.6671, 29.384) (12.6385, 29.7635) (12.6008, 30.1422) (12.5682, 30.3938) (12.5519, 30.5196) knots 0 0 0 0 0.031256 0.062512 0.093767 0.125023 0.156279 0.187534 0.218789 0.250044 0.281299 0.312553 0.343805 0.375056 0.390675 0.406289 0.421901 0.43751 0.453121 0.460935 0.468748 0.476559 0.484372 0.5 0.515628 0.523441 0.531252 0.539065 0.546879 0.56249 0.578099 0.593711 0.609325 0.624944 0.656195 0.687447 0.718701 0.749956 0.781211 0.812466 0.843721 0.874977 0.906233 0.937488 0.968744 1 1 1 1 projected
  arc A25 (12.5519, 30.5196) -> (10.843, 31.1678) centre (0, 0) ccw projected
  constraints: 2 horizontal alignment, 24 other
extrude "Extrusion3" cut sketch "Esquisse2" against normal blind 14
sketch "Esquisse3" plane through (0, 0, -14) normal (0, 0, 1) x (1, 0, 0)
  arc A0 (0, 5) -> (5, 0) centre (0, 0) ccw construction
  line L0 (0, 0) -> (-5, 0) construction
  line L1 (0, 0) -> (-2.9389, 4.0451) construction
  line L2 (-18.3521, 30.971) -> (-11.8455, 22.0155)
  arc A1 (-35.8922, -2.7843) -> (-18.3521, 30.971) centre (0, 0) ccw
  arc A2 (-24.8445, -2.7843) -> (-11.8455, 22.0155) centre (0, 0) ccw
  line L3 (0, 0) -> (-5, 0)
  line L4 (-24.8445, -2.7843) -> (-35.8922, -2.7843)
  line L5 (0, 0) -> (-2.9389, 4.0451)
  line L6 (-11.8455, 22.0155) -> (-18.3521, 30.971)
  line L7 (0, 0) -> (7.75, 0)
  circle A3 centre (7.75, 0) radius 1.15
  line L8 (8.8758, -1.95) -> (6.6242, -1.95)
  line L9 (6.6242, -1.95) -> (5.4983, 0)
  line L10 (5.4983, 0) -> (6.6242, 1.95)
  line L11 (6.6242, 1.95) -> (8.8758, 1.95)
  line L12 (8.8758, 1.95) -> (10.0017, 0)
  line L13 (10.0017, 0) -> (8.8758, -1.95)
  line L14 (0, 0) -> (0, 7.75)
  circle A4 centre (0, 7.75) radius 1.15
  line L15 (1.95, 8.8758) -> (1.95, 6.6242)
  line L16 (1.95, 6.6242) -> (0, 5.4983)
  line L17 (0, 5.4983) -> (-1.95, 6.6242)
  line L18 (-1.95, 6.6242) -> (-1.95, 8.8758)
  line L19 (-1.95, 8.8758) -> (0, 10.0017)
  line L20 (0, 10.0017) -> (1.95, 8.8758)
  line L21 (0, 0) -> (-7.75, 0)
  circle A5 centre (-7.75, 0) radius 1.15
  line L22 (-8.8758, 1.95) -> (-6.6242, 1.95)
  line L23 (-6.6242, 1.95) -> (-5.4983, 0)
  line L24 (-5.4983, 0) -> (-6.6242, -1.95)
  line L25 (-6.6242, -1.95) -> (-8.8758, -1.95)
  line L26 (-8.8758, -1.95) -> (-10.0017, 0)
  line L27 (-10.0017, 0) -> (-8.8758, 1.95)
  line L28 (0, 0) -> (0, -7.75)
  circle A6 centre (0, -7.75) radius 1.15
  line L29 (-1.95, -8.8758) -> (-1.95, -6.6242)
  line L30 (-1.95, -6.6242) -> (0, -5.4983)
  line L31 (0, -5.4983) -> (1.95, -6.6242)
  line L32 (1.95, -6.6242) -> (1.95, -8.8758)
  line L33 (1.95, -8.8758) -> (0, -10.0017)
  line L34 (0, -10.0017) -> (-1.95, -8.8758)
  dimension "d9" = 10
  dimension "d10" = 54
  dimension "d11" = 36
  dimension "d13" = 50
  dimension "d17" = 7.75
  dimension "d18" = 2.3
  dimension "d19" = 3.9
  dimension "d20" = 360
  constraints: 70 end point, 12 coincident, 8 point on circle, 7 centre point, 4 horizontal, 2 point on line, 86 other
  measures "d9" diameter of A0
  measures "d10" angle of L1 L0
  measures "d11" distance of L0.start L4.end
  measures "d13" diameter of A2
  measures "d17" distance of L7.start L7.end
  measures "d18" diameter of A3
  measures "d19" distance between parallel lines of L8 L11
sketch "Esquisse4" plane through (0, 0, -14) normal (0, 0, 1) x (1, 0, 0)
  arc A0 (-17.006, -3.5568) -> (-5.8798, 13.5862) centre (-14.8586, 7.2316) ccw
  arc A1 (-24.8445, -2.7843) -> (-11.8455, 22.0155) centre (0, 0) ccw projected
  line L0 (-24.8445, -2.7843) -> (-14.8586, -3.7684)
  line L1 (-11.8455, 22.0155) -> (-5.8798, 13.5862)
  arc A2 (-24.8445, -2.7843) -> (-11.8455, 22.0155) centre (0, 0) ccw
  point P0 (0, 0)
  dimension "d24" = 22
  constraints: 5 point on circle, 4 end point, 2 centre point, 1 coincident, 1 concentric, 1 point on line, 1 tangent
  measures "d24" diameter of A0
extrude "Extrusion5" cut sketch "Esquisse4" against normal blind 10 contours A0 L1 A1 L0
sketch "Esquisse5" plane through (0, 0, -14) normal (0, 0, 1) x (1, 0, 0)
  point P0 (0, 0)
extrude "Extrusion6" cut sketch "Esquisse3" against normal blind 10 contours A1 L4 A2 L2
sketch "Esquisse7" plane through (0, 0, -14) normal (0, 0, 1) x (1, 0, 0)
  point P0 (0, 0)
sketch "Esquisse8" plane through (0, 0, -14) normal (0, 0, 1) x (1, 0, 0)
  circle A0 centre (-14.8586, 7.2316) radius 11
  line L0 (-14.8586, 7.2316) -> (-7.1086, 7.2316)
  circle A1 centre (-7.1086, 7.2316) radius 1.15
  line L1 (-6.5834, 5.042) -> (-8.7422, 5.6819)
  line L2 (-8.7422, 5.6819) -> (-9.2674, 7.8715)
  line L3 (-9.2674, 7.8715) -> (-7.6338, 9.4211)
  line L4 (-7.6338, 9.4211) -> (-5.475, 8.7812)
  line L5 (-5.475, 8.7812) -> (-4.9498, 6.5916)
  line L6 (-4.9498, 6.5916) -> (-6.5834, 5.042)
  line L7 (-14.8586, 7.2316) -> (-14.8586, 14.9816)
  circle A2 centre (-14.8586, 14.9816) radius 1.15
  line L8 (-12.6691, 15.5068) -> (-13.309, 13.348)
  line L9 (-13.309, 13.348) -> (-15.4985, 12.8227)
  line L10 (-15.4985, 12.8227) -> (-17.0482, 14.4563)
  line L11 (-17.0482, 14.4563) -> (-16.4083, 16.6151)
  line L12 (-16.4083, 16.6151) -> (-14.2187, 17.1404)
  line L13 (-14.2187, 17.1404) -> (-12.6691, 15.5068)
  line L14 (-14.8586, 7.2316) -> (-22.6086, 7.2316)
  circle A3 centre (-22.6086, 7.2316) radius 1.15
  line L15 (-23.1338, 9.4211) -> (-20.975, 8.7812)
  line L16 (-20.975, 8.7812) -> (-20.4498, 6.5916)
  line L17 (-20.4498, 6.5916) -> (-22.0834, 5.042)
  line L18 (-22.0834, 5.042) -> (-24.2422, 5.6819)
  line L19 (-24.2422, 5.6819) -> (-24.7674, 7.8715)
  line L20 (-24.7674, 7.8715) -> (-23.1338, 9.4211)
  line L21 (-14.8586, 7.2316) -> (-14.8586, -0.5184)
  circle A4 centre (-14.8586, -0.5184) radius 1.15
  line L22 (-17.0482, -1.0437) -> (-16.4083, 1.1151)
  line L23 (-16.4083, 1.1151) -> (-14.2187, 1.6404)
  line L24 (-14.2187, 1.6404) -> (-12.6691, 0.0068)
  line L25 (-12.6691, 0.0068) -> (-13.309, -2.152)
  line L26 (-13.309, -2.152) -> (-15.4985, -2.6773)
  line L27 (-15.4985, -2.6773) -> (-17.0482, -1.0437)
  line L28 (0, 0) -> (7.75, 0)
  circle A5 centre (7.75, 0) radius 1.15
  line L29 (8.8758, -1.95) -> (6.6242, -1.95)
  line L30 (6.6242, -1.95) -> (5.4983, 0)
  line L31 (5.4983, 0) -> (6.6242, 1.95)
  line L32 (6.6242, 1.95) -> (8.8758, 1.95)
  line L33 (8.8758, 1.95) -> (10.0017, 0)
  line L34 (10.0017, 0) -> (8.8758, -1.95)
  line L35 (0, 0) -> (0, 7.75)
  circle A6 centre (0, 7.75) radius 1.15
  line L36 (1.95, 8.8758) -> (1.95, 6.6242)
  line L37 (1.95, 6.6242) -> (0, 5.4983)
  line L38 (0, 5.4983) -> (-1.95, 6.6242)
  line L39 (-1.95, 6.6242) -> (-1.95, 8.8758)
  line L40 (-1.95, 8.8758) -> (0, 10.0017)
  line L41 (0, 10.0017) -> (1.95, 8.8758)
  line L42 (0, 0) -> (-7.75, 0)
  circle A7 centre (-7.75, 0) radius 1.15
  line L43 (-8.8758, 1.95) -> (-6.6242, 1.95)
  line L44 (-6.6242, 1.95) -> (-5.4983, 0)
  line L45 (-5.4983, 0) -> (-6.6242, -1.95)
  line L46 (-6.6242, -1.95) -> (-8.8758, -1.95)
  line L47 (-8.8758, -1.95) -> (-10.0017, 0)
  line L48 (-10.0017, 0) -> (-8.8758, 1.95)
  line L49 (0, 0) -> (0, -7.75)
  circle A8 centre (0, -7.75) radius 1.15
  line L50 (-1.95, -8.8758) -> (-1.95, -6.6242)
  line L51 (-1.95, -6.6242) -> (0, -5.4983)
  line L52 (0, -5.4983) -> (1.95, -6.6242)
  line L53 (1.95, -6.6242) -> (1.95, -8.8758)
  line L54 (1.95, -8.8758) -> (0, -10.0017)
  line L55 (0, -10.0017) -> (-1.95, -8.8758)
  arc A9 (-17.006, -3.5568) -> (-5.8798, 13.5862) centre (-14.8586, 7.2316) ccw projected
  circle A10 centre (-14.8586, 7.2316) radius 1.35
  dimension "d51" = 22
  dimension "d52" = 7.75
  dimension "d53" = 2.3
  dimension "d54" = 3.9
  dimension "d55" = 360
  dimension "d59" = 7.75
  dimension "d60" = 2.3
  dimension "d61" = 3.9
  dimension "d62" = 360
  dimension "d63" = 2.7
  constraints: 112 end point, 20 coincident, 10 centre point, 2 horizontal, 172 other
  measures "d51" diameter of A0
  measures "d52" distance of L0.start L0.end
  measures "d53" diameter of A1
  measures "d54" distance between parallel lines of L1 L4
  measures "d59" distance of L28.start L28.end
  measures "d60" diameter of A5
  measures "d61" distance between parallel lines of L29 L32
  measures "d63" diameter of A10
extrude "Extrusion7" cut sketch "Esquisse8" against normal blind 10 contours L7 A10 L0 | L14 A10 L7 | L21 A10 L14 | L0 A10 L21 | A1 | A2 | A3 | A4
sketch "Esquisse9" plane through (0, 0, -14) normal (0, 0, 1) x (1, 0, 0)
  point P0 (0, 0)
equation "\"d0\" = Largeur_de_la_face"
equation "\"Module\" = 2.25"
equation "\"Angle_de_pression\" = 20deg"
equation "\"Unité_Dégagement_de_contour\" = 0.25"
equation "\"Diamètre_de_la_tête\" = 66"
equation "\"Diamètre_de_la_racine\" = 55.89242"
equation "\"Diamètre_de_la_base\" = 57.08633"
equation "\"Diamètre_primitif\" = 60.75"
equation "\"Largeur_de_la_face\" = 20"
equation "\"Angle_hélice\" = 0"
equation "\"Unité_Correction\" = 0.170539"
equation "\"Unité_Modification_de_la_saillie\" = 0.003872"
equation "\"Pas_circulaire\" = 7.068583"
equation "\"Unité_Décalage_de_jeu_entre_dents\" = 0"
equation "\"Décalage_total_des_outils\" = 0.38371"
equation "\"Est_interne\" = 0"
